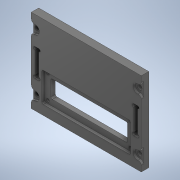
# Autodesk Inventor part: Cockpit_horizontal_frame_05
Saved by Autodesk Inventor 2020.4 (Build 244396000, 396)
## iProperties
Created: 2021-08-14
Part Number: Cockpit_horizontal_frame_05
Material: アセタール樹脂、黒
Document SubType Name: Modeling
Designer: Masato Kubotera
Density: 1.425 g/cm^3
Appearance: 滑らか - 黒
Mass: 37.8231 g
Surface Area: 126.929 cm^2
Volume: 26.5425 cm^3
Description: POM T5
Author: Masato Kubotera
Title: Cockpit_horizontal_frame_05
Autodesk Inventor part; units mm, degrees
ref_plane "YZ Plane" through (0, 0, 0) normal (1, 0, 0) x (0, 1, 0)
ref_plane "XZ Plane" through (0, 0, 0) normal (0, 1, 0) x (-1, 0, 0)
ref_plane "XY Plane" through (0, 0, 0) normal (0, 0, 1) x (1, 0, 0)
sketch "スケッチ1" plane through (0, 0, 0) normal (0, 0, 1) x (1, 0, 0)
  line L0 (37.25, 28.25) -> (37.25, 23.75)
  line L1 (37.25, -28.25) -> (-37.25, -28.25)
  line L2 (-37.25, -28.25) -> (-37.25, -11.5167)
  line L3 (-37.25, 28.25) -> (37.25, -28.25) construction
  line L4 (37.25, 28.25) -> (-37.25, -28.25) construction
  line L5 (0, 28.25) -> (0, -28.25) construction
  line L6 (-37.25, 11.5167) -> (-37.25, 28.25)
  line L7 (-37.25, -11.5167) -> (-37.25, 11.5167)
  line L8 (37.25, 11.5167) -> (37.25, -11.5167)
  line L9 (37.25, -11.5167) -> (37.25, -28.25)
  line L10 (-37.25, 0) -> (37.25, 0) construction
  line L11 (37.25, 23.75) -> (37.25, 11.5167)
  line L12 (-30, -1.75) -> (30, -1.75) construction
  line L13 (30, -1.75) -> (30, -21.75) construction
  line L14 (30, -21.75) -> (-30, -21.75) construction
  line L15 (-30, -21.75) -> (-30, -1.75) construction
  line L16 (-30, -1.75) -> (30, -21.75) construction
  line L17 (30, -1.75) -> (-30, -21.75) construction
  circle A0 centre (-28, -3.75) radius 1.05
  line L18 (30, -11.75) -> (-30, -11.75) construction
  circle A1 centre (-28, -19.75) radius 1.05
  circle A2 centre (28, -3.75) radius 1.05
  circle A3 centre (28, -19.75) radius 1.05
  line L19 (-30.05, -1.7) -> (30.05, -1.7)
  line L20 (30.05, -1.7) -> (30.05, -21.8)
  line L21 (30.05, -21.8) -> (-30.05, -21.8)
  line L22 (-30.05, -21.8) -> (-30.05, -1.7)
  line L23 (-30.05, -1.7) -> (30.05, -21.8) construction
  line L24 (30.05, -1.7) -> (-30.05, -21.8) construction
  line L25 (-26, -5.75) -> (26, -5.75)
  line L26 (26, -5.75) -> (26, -17.75)
  line L27 (26, -17.75) -> (-26, -17.75)
  line L28 (-26, -17.75) -> (-26, -5.75)
  line L29 (-26, -5.75) -> (26, -17.75) construction
  line L30 (26, -5.75) -> (-26, -17.75) construction
  line L31 (-34.75, 9.4167) -> (-32.25, 9.4167) construction
  line L32 (-32.25, 9.4167) -> (-32.25, -9.4167) construction
  line L33 (-32.25, -9.4167) -> (-34.75, -9.4167) construction
  line L34 (-34.75, -9.4167) -> (-34.75, 9.4167) construction
  line L35 (-34.75, 9.4167) -> (-32.25, -9.4167) construction
  line L36 (-32.25, 9.4167) -> (-34.75, -9.4167) construction
  line L37 (-34.76, 9.4267) -> (-32.24, 9.4267)
  line L38 (-32.24, 9.4267) -> (-32.24, 7.3267) construction
  line L39 (-32.24, -9.4267) -> (-34.76, -9.4267)
  line L40 (-34.76, -9.4267) -> (-34.76, -7.3267) construction
  line L41 (-34.76, 9.4267) -> (-32.24, -9.4267) construction
  line L42 (-32.24, 9.4267) -> (-34.76, -9.4267) construction
  arc A4 (-34.76, 9.4267) -> (-34.76, 7.3267) centre (-34.76, 8.3767) ccw
  line L43 (-33.5, 9.4167) -> (-33.5, -9.4167) construction
  line L44 (-34.75, 0) -> (-32.25, 0) construction
  arc A5 (-32.24, 7.3267) -> (-32.24, 9.4267) centre (-32.24, 8.3767) ccw
  arc A6 (-34.76, -7.3267) -> (-34.76, -9.4267) centre (-34.76, -8.3767) ccw
  arc A7 (-32.24, -9.4267) -> (-32.24, -7.3267) centre (-32.24, -8.3767) ccw
  line L45 (-34.76, 7.3267) -> (-34.76, 9.4267) construction
  line L46 (-32.24, 7.3267) -> (-32.24, -7.3267)
  line L47 (-34.76, -7.3267) -> (-34.76, 7.3267)
  line L48 (-32.24, -7.3267) -> (-32.24, -9.4267) construction
  line L49 (34.75, 9.4167) -> (32.25, 9.4167) construction
  line L50 (32.25, 9.4167) -> (32.25, -9.4167) construction
  line L51 (32.25, -9.4167) -> (34.75, -9.4167) construction
  line L52 (34.75, -9.4167) -> (34.75, 9.4167) construction
  line L53 (34.75, 9.4167) -> (32.25, -9.4167) construction
  line L54 (32.25, 9.4167) -> (34.75, -9.4167) construction
  line L55 (34.76, 9.4267) -> (32.24, 9.4267)
  line L56 (32.24, 9.4267) -> (32.24, 7.3267) construction
  line L57 (32.24, -9.4267) -> (34.76, -9.4267)
  line L58 (34.76, -9.4267) -> (34.76, -7.3267) construction
  line L59 (34.76, 9.4267) -> (32.24, -9.4267) construction
  line L60 (32.24, 9.4267) -> (34.76, -9.4267) construction
  arc A8 (34.76, 7.3267) -> (34.76, 9.4267) centre (34.76, 8.3767) ccw
  line L61 (33.5, 9.4167) -> (33.5, -9.4167) construction
  line L62 (34.75, 0) -> (32.25, 0) construction
  arc A9 (32.24, 9.4267) -> (32.24, 7.3267) centre (32.24, 8.3767) ccw
  arc A10 (34.76, -9.4267) -> (34.76, -7.3267) centre (34.76, -8.3767) ccw
  arc A11 (32.24, -7.3267) -> (32.24, -9.4267) centre (32.24, -8.3767) ccw
  line L63 (34.76, 7.3267) -> (34.76, 9.4267) construction
  line L64 (32.24, 7.3267) -> (32.24, -7.3267)
  line L65 (34.76, -7.3267) -> (34.76, 7.3267)
  line L66 (32.24, -7.3267) -> (32.24, -9.4267) construction
  circle A12 centre (-34.75, 19.4167) radius 1.55
  circle A13 centre (-34.75, 19.4167) radius 3
  circle A14 centre (34.75, 19.4167) radius 1.55
  circle A15 centre (34.75, 19.4167) radius 3
  circle A16 centre (-34.75, -19.4167) radius 3
  circle A17 centre (34.75, -19.4167) radius 3
  circle A18 centre (34.75, -19.4167) radius 1.55
  circle A19 centre (-34.75, -19.4167) radius 1.55
  line L67 (37.25, 28.25) -> (-37.25, 28.25)
  point P0 (0, 0)
  point P1 (0, 0)
  point P2 (0, 0)
  point P3 (0, 0)
  point P4 (0, -11.75)
  point P5 (-33.5, 0)
  point P6 (-33.5, 0)
  point P7 (-33.5, 0)
  point P8 (33.5, 0)
  point P9 (33.5, 0)
  point P10 (33.5, 0)
  point P11 (-33.5, 0)
  point P12 (37.25, 17.7584)
  point P13 (37.25, 21.075)
  point P14 (37.25, -21.075)
  point P15 (37.25, -17.7584)
  point P16 (-37.25, -17.7584)
  point P17 (-37.25, -21.075)
  point P18 (-37.25, 21.075)
  point P19 (-37.25, 17.7584)
  point P20 (-37.25, 21.075)
  dimension "d96" = 6
  dimension "d69" = 60
  dimension "d70" = 20
  dimension "d71" = 2
  dimension "d72" = 2
  dimension "d73" = 2.1
  dimension "d75" = 0.05
  dimension "d76" = 0.05
  dimension "d80" = 4
  dimension "d81" = 4
  dimension "d82" = 2.5
  dimension "d83" = 18.8333
  dimension "d84" = 1.05
  dimension "d87" = 0.01
  dimension "d88" = 0.01
  dimension "d89" = 64.5
  dimension "d95" = 3.1
  dimension "d97" = 10
  dimension "d100" = 11.75
  dimension "d102" = 2.5
  dimension "d103" = 5
  dimension "d109" = 56.5
  constraints: 136 end point, 41 symmetric about line, 36 midpoint, 30 parallel, 19 centre point, 16 point on circle, 8 perpendicular, 6 horizontal, 5 point on line, 3 coincident, 19 other
  measures "d69" distance of L13.end L14.end
  measures "d70" distance of L12.end L13.end
  measures "d71" horizontal distance of A0.centre L12.start
  measures "d72" horizontal distance of L12.start A0.centre
  measures "d73" diameter of A0
  measures "d75" horizontal distance of L19.start L12.start
  measures "d76" horizontal distance of L12.start L19.start
  measures "d80" horizontal distance of L25.start L12.start
  measures "d81" horizontal distance of L25.start L12.start
  measures "d82" distance of L32.end L33.end
  measures "d83" distance of L31.end L32.end
  measures "d84" radius of A4
  measures "d87" distance between parallel lines of L31 L37
  measures "d88" distance between parallel lines of L34 L47
  measures "d89" distance between parallel lines of L32 L50
  measures "d95" diameter of A12
  measures "d97" distance from line of A12.centre L31
  measures "d100" distance of point (0, -11.75) point (0, 0)
  measures "d102" distance from line of L32 A12.centre
  measures "d103" distance from line of L32 L3.start
  measures "d109" distance of L1.start L0.start
extrude "押し出し1" add sketch "スケッチ1" along normal blind 5 contours L0 L11 A15 L8 L9 A17 L1 L2 A16 L7 L6 A13 L67
extrude "押し出し2" add sketch "スケッチ1" along normal blind 3 contours L19 L20 L21 L22
fillet "フィレット1" radius 1 8 edges at (-30.05, -1.7, 4) (-30.05, -21.8, 4) (30.05, -21.8, 4) (30.05, -1.7, 4) (-26, -5.75, 1.5) (-26, -17.75, 1.5) (26, -5.75, 1.5) (26, -17.75, 1.5)
extrude "押し出し3" add sketch "スケッチ1" along normal blind 3.5 contours L11 A15 | A13 L6 | L9 A17 | A16 L2 picked at (36.9333, 19.4167) picked at (-36.9333, 19.4167) picked at (36.9333, -19.4167) picked at (-36.9333, -19.4167)
fillet "フィレット5" radius 2 8 edges at (-37.25, -21.075, 4.25) (37.25, -21.075, 4.25) (37.25, -17.7584, 4.25) (-37.25, -17.7584, 4.25) (-37.25, 17.7584, 4.25) (37.25, 17.7584, 4.25) (37.25, 21.075, 4.25) (-37.25, 21.075, 4.25)
